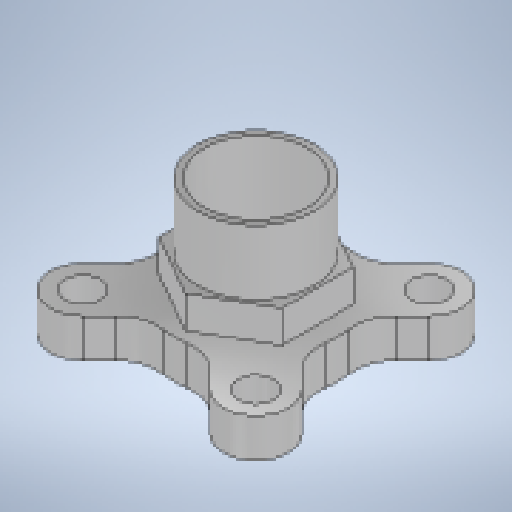
# Autodesk Inventor part: Custom Base
Saved by Autodesk Inventor 2023.4 (Build 274418000, 418)
## iProperties
Created: 2024-04-22
Part Number: Custom Base
Material: Aluminum 6061
Document SubType Name: Modeling
Designer: Nathan Cai
Density: 2.7 g/cm^3
Appearance: Aluminum - Flat
Author: Nathan Cai
Autodesk Inventor part; units mm, degrees
ref_plane "YZ Plane" through (0, 0, 0) normal (1, 0, 0) x (0, 1, 0)
ref_plane "XZ Plane" through (0, 0, 0) normal (0, 1, 0) x (-1, 0, 0)
ref_plane "XY Plane" through (0, 0, 0) normal (0, 0, 1) x (1, 0, 0)
sketch "Sketch1" plane through (0, 0, 0) normal (0, 1, 0) x (-1, 0, 0)
  circle A0 centre (0, 0) radius 9.5 construction
  circle A1 centre (0, 0) radius 9.5 construction
  line L0 (0, 0) -> (9.5, 0) construction
  line L1 (0, 0) -> (6.7175, -6.7175) construction
  circle A2 centre (6.7175, -6.7175) radius 1.375
  line L2 (0, 0) -> (6.7175, 6.7175) construction
  circle A3 centre (6.7175, 6.7175) radius 1.375
  circle A4 centre (-6.7175, -6.7175) radius 1.375
  circle A5 centre (-6.7175, 6.7175) radius 1.375
  circle A6 centre (0, 0) radius 4
  line L3 (-6.7175, -6.7175) -> (6.7175, 6.7175) construction
  arc A7 (-8.4853, -4.9497) -> (-4.9497, -8.4853) centre (-6.7175, -6.7175) ccw
  arc A8 (8.4853, 4.9497) -> (4.9497, 8.4853) centre (6.7175, 6.7175) ccw
  line L4 (-6.7175, 6.7175) -> (6.7175, -6.7175) construction
  arc A9 (-4.9497, 8.4853) -> (-8.4853, 4.9497) centre (-6.7175, 6.7175) ccw
  arc A10 (4.9497, -8.4853) -> (8.4853, -4.9497) centre (6.7175, -6.7175) ccw
  line L5 (4.7625, -2.7496) -> (0, -5.4993)
  line L6 (0, -5.4993) -> (-4.7625, -2.7496)
  line L7 (-4.7625, -2.7496) -> (-4.7625, 2.7496)
  line L8 (-4.7625, 2.7496) -> (0, 5.4993)
  line L9 (0, 5.4993) -> (4.7625, 2.7496)
  line L10 (4.7625, 2.7496) -> (4.7625, -2.7496)
  line L11 (-4.9497, -8.4853) -> (-1.245, -4.7805)
  line L12 (4.7625, 1.227) -> (8.4853, 4.9497)
  line L13 (4.9497, 8.4853) -> (1.245, 4.7805)
  line L14 (-4.7625, -1.227) -> (-8.4853, -4.9497)
  line L15 (-8.4853, 4.9497) -> (-4.7625, 1.227)
  line L16 (1.245, -4.7805) -> (4.9497, -8.4853)
  line L17 (8.4853, -4.9497) -> (4.7625, -1.227)
  line L18 (-1.245, 4.7805) -> (-4.9497, 8.4853)
  circle A11 centre (0, 0) radius 4.5
  circle A12 centre (0, 0) radius 6.35
  point P0 (4.7625, 0)
  point P1 (-2.3597, -5.8953)
  point P2 (2.3597, -5.8953)
  point P3 (-5.8953, 2.3597)
  point P4 (-5.8953, -2.3597)
  point P5 (2.3597, 5.8953)
  point P6 (-2.3597, 5.8953)
  point P7 (5.8953, 2.3597)
  point P8 (5.8953, -2.3597)
  dimension "d1" = 19
  dimension "d0" = 19
  dimension "d2" = 2.75
  dimension "d3" = 45
  dimension "d4" = 2.75
  dimension "d7" = 360
  dimension "d9" = 8
  dimension "d10" = 5
  dimension "d11" = 5
  dimension "d13" = 9.525
  dimension "d16" = 9
  dimension "d22" = 12.7
  constraints: 42 end point, 16 tangent, 12 centre point, 10 point on circle, 9 point on line, 8 coincident, 8 parallel, 3 midpoint, 2 collinear, 1 horizontal, 1 perpendicular, 25 other
  measures "d0" diameter of A0
  measures "d2" diameter of A2
  measures "d3" angle of L0 L1
  measures "d4" diameter of A3
  measures "d9" diameter of A6
  measures "d10" diameter of A8
  measures "d11" diameter of A10
  measures "d13" distance between parallel lines of L7 L10
  measures "d16" diameter of A11
  measures "d22" diameter of A12
extrude "Extrusion1" add sketch "Sketch1" along normal blind 3 contours L14 A12 L11 A7 | A12 L15 L7 L14 | L14 L7 L6 L11 A12 | L11 L6 L5 L16 A12 | L7 L8 L9 L10 L5 L6 | A12 L18 L8 L7 L15 | L15 A9 L18 A12 | A12 L17 A10 L16 | L16 L5 L10 L17 A12 | A12 L13 L9 L8 L18 | L17 L10 L12 A12 | A12 L12 L10 L9 L13 | L13 A8 L12 A12 | A11
extrude "Extrusion2" add sketch "Sketch1" along normal blind 5.5 contours L7 L8 L9 L10 L5 L6 | A11
extrude "Extrusion3" add sketch "Sketch1" along normal blind 10.5 contours A11
fillet "Fillet1" radius 3.175 8 edges at (2.3597, 1.5, -5.8953) (-2.3597, 1.5, -5.8953) (-5.8953, 1.5, 2.3597) (-5.8953, 1.5, -2.3597) (-2.3597, 1.5, 5.8953) (2.3597, 1.5, 5.8953) (5.8953, 1.5, -2.3597) (5.8953, 1.5, 2.3597)
equation "\"d1\" = d0"
equation "\"d2\" = d4"
body "Solid1"
